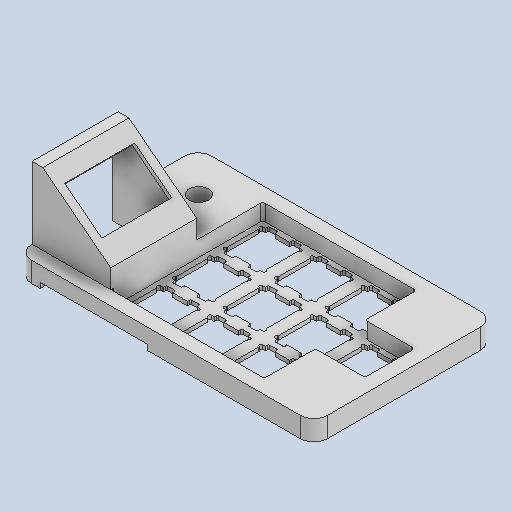
# Autodesk Inventor part: q
Saved by Autodesk Inventor 2025.2 (Build 292293000, 293)
## iProperties
Created: 2024-03-08
Part Number: q
Material: Generic
Document SubType Name: Modeling
Designer: mirun
Density: 1 g/cm^3
Appearance: Default
Author: mirun
Autodesk Inventor part; units mm, degrees
(part 1 of 2)
ref_plane "YZ Plane" through (0, 0, 0) normal (1, 0, 0) x (0, 1, 0)
sketch "Sketch1" plane through (0, 0, 0) normal (0, 1, 0) x (-1, 0, 0)
  line L0 (7.25, 5.8376) -> (7.25, -5.8376)
  line L1 (-7.25, -5.8376) -> (-7.25, 5.8376)
  line L2 (-7.25, 7.25) -> (7.25, -7.25) construction
  line L3 (7.25, 7.25) -> (-7.25, -7.25) construction
  line L4 (6.25, 7.25) -> (2.75, 7.25) construction
  line L5 (2.75, 7.35) -> (2.75, 7.95)
  line L6 (3.25, 8.45) -> (5.75, 8.45)
  line L7 (6.25, 7.95) -> (6.25, 7.35)
  arc A0 (7.4265, 6.0765) -> (7.25, 7.25) centre (7.25, 6.65) ccw
  line L8 (-7.25, 7.25) -> (2.65, 7.25)
  line L9 (6.35, 7.25) -> (7.25, 7.25)
  arc A1 (6.25, 7.35) -> (6.35, 7.25) centre (6.35, 7.35) ccw
  arc A2 (2.65, 7.25) -> (2.75, 7.35) centre (2.65, 7.35) ccw
  arc A3 (6.25, 7.95) -> (5.75, 8.45) centre (5.75, 7.95) ccw
  arc A4 (3.25, 8.45) -> (2.75, 7.95) centre (3.25, 7.95) ccw
  arc A5 (7.4265, 6.0765) -> (7.25, 5.8376) centre (7.5, 5.8376) ccw
  line L10 (0, 0) -> (3.0164, 0)
  line L11 (0, 0) -> (0, -4.9825)
  arc A6 (7.25, -5.8376) -> (7.4265, -6.0765) centre (7.5, -5.8376) ccw
  arc A7 (7.25, -7.25) -> (7.4265, -6.0765) centre (7.25, -6.65) ccw
  line L12 (6.35, -7.25) -> (7.25, -7.25)
  line L13 (7.25, -7.25) -> (-7.25, 7.25) construction
  arc A8 (6.35, -7.25) -> (6.25, -7.35) centre (6.35, -7.35) ccw
  line L14 (6.25, -7.95) -> (6.25, -7.35)
  arc A9 (5.75, -8.45) -> (6.25, -7.95) centre (5.75, -7.95) ccw
  line L15 (6.25, -7.25) -> (2.75, -7.25) construction
  line L16 (3.25, -8.45) -> (5.75, -8.45)
  arc A10 (2.75, -7.35) -> (2.65, -7.25) centre (2.65, -7.35) ccw
  line L17 (2.75, -7.35) -> (2.75, -7.95)
  arc A11 (2.75, -7.95) -> (3.25, -8.45) centre (3.25, -7.95) ccw
  line L18 (7.25, -7.25) -> (6.35, -7.25)
  arc A12 (-6.35, 7.25) -> (-6.25, 7.35) centre (-6.35, 7.35) ccw
  line L19 (-6.35, 7.25) -> (-7.25, 7.25)
  arc A13 (-7.25, 5.8376) -> (-7.4265, 6.0765) centre (-7.5, 5.8376) ccw
  arc A14 (-7.25, 7.25) -> (-7.4265, 6.0765) centre (-7.25, 6.65) ccw
  line L20 (-6.25, 7.95) -> (-6.25, 7.35)
  line L21 (-3.25, 8.45) -> (-5.75, 8.45)
  line L22 (-2.75, 7.35) -> (-2.75, 7.95)
  line L23 (-6.25, 7.25) -> (-2.75, 7.25) construction
  arc A15 (-2.75, 7.95) -> (-3.25, 8.45) centre (-3.25, 7.95) ccw
  arc A16 (-2.75, 7.35) -> (-2.65, 7.25) centre (-2.65, 7.35) ccw
  arc A17 (-5.75, 8.45) -> (-6.25, 7.95) centre (-5.75, 7.95) ccw
  line L24 (-7.25, -7.25) -> (7.25, 7.25) construction
  line L25 (-6.25, -7.25) -> (-2.75, -7.25) construction
  arc A18 (-6.25, -7.35) -> (-6.35, -7.25) centre (-6.35, -7.35) ccw
  line L26 (-2.75, -7.35) -> (-2.75, -7.95)
  line L27 (-6.25, -7.95) -> (-6.25, -7.35)
  arc A19 (-3.25, -8.45) -> (-2.75, -7.95) centre (-3.25, -7.95) ccw
  line L28 (-3.25, -8.45) -> (-5.75, -8.45)
  arc A20 (-6.25, -7.95) -> (-5.75, -8.45) centre (-5.75, -7.95) ccw
  line L29 (-6.35, -7.25) -> (-7.25, -7.25)
  line L30 (-7.25, -7.25) -> (-6.35, -7.25)
  arc A21 (-7.4265, -6.0765) -> (-7.25, -5.8376) centre (-7.5, -5.8376) ccw
  arc A22 (-7.4265, -6.0765) -> (-7.25, -7.25) centre (-7.25, -6.65) ccw
  arc A23 (-2.65, -7.25) -> (-2.75, -7.35) centre (-2.65, -7.35) ccw
  line L31 (2.65, -7.25) -> (-2.65, -7.25)
  line L32 (-6.35, -7.25) -> (-7.25, -7.25)
  line L33 (-12.65, 7.25) -> (-11.75, 7.25)
  arc A24 (-11.5735, 6.0765) -> (-11.75, 5.8376) centre (-11.5, 5.8376) ccw
  arc A25 (-11.5735, 6.0765) -> (-11.75, 7.25) centre (-11.75, 6.65) ccw
  arc A26 (-12.75, 7.35) -> (-12.65, 7.25) centre (-12.65, 7.35) ccw
  line L34 (-11.75, 5.8376) -> (-11.75, -5.8376)
  line L35 (-26.25, -5.8376) -> (-26.25, 5.8376)
  line L36 (-26.25, 7.25) -> (-11.75, -7.25) construction
  line L37 (-11.75, 7.25) -> (-26.25, -7.25) construction
  line L38 (-12.75, 7.25) -> (-16.25, 7.25) construction
  line L39 (-19, 0) -> (-15.9836, 0)
  line L40 (-25.25, 7.25) -> (-21.75, 7.25) construction
  line L41 (-26.25, 7.25) -> (-16.35, 7.25)
  line L42 (-25.35, 7.25) -> (-26.25, 7.25)
  line L43 (-11.75, -7.25) -> (-26.25, 7.25) construction
  line L44 (-26.25, -7.25) -> (-11.75, 7.25) construction
  line L45 (-19, 0) -> (-19, -4.9825)
  line L46 (-12.75, 7.95) -> (-12.75, 7.35)
  arc A27 (-12.75, 7.95) -> (-13.25, 8.45) centre (-13.25, 7.95) ccw
  line L47 (-15.75, 8.45) -> (-13.25, 8.45)
  arc A28 (-15.75, 8.45) -> (-16.25, 7.95) centre (-15.75, 7.95) ccw
  line L48 (-16.25, 7.35) -> (-16.25, 7.95)
  arc A29 (-16.35, 7.25) -> (-16.25, 7.35) centre (-16.35, 7.35) ccw
  arc A30 (-12.65, -7.25) -> (-12.75, -7.35) centre (-12.65, -7.35) ccw
  line L49 (-12.75, -7.25) -> (-16.25, -7.25) construction
  arc A31 (-16.25, -7.35) -> (-16.35, -7.25) centre (-16.35, -7.35) ccw
  line L50 (-16.25, -7.35) -> (-16.25, -7.95)
  line L51 (-16.35, -7.25) -> (-21.65, -7.25)
  arc A32 (-21.65, -7.25) -> (-21.75, -7.35) centre (-21.65, -7.35) ccw
  line L52 (-11.75, -7.25) -> (-12.65, -7.25)
  arc A33 (-11.75, -5.8376) -> (-11.5735, -6.0765) centre (-11.5, -5.8376) ccw
  arc A34 (-11.75, -7.25) -> (-11.5735, -6.0765) centre (-11.75, -6.65) ccw
  line L53 (-12.65, -7.25) -> (-11.75, -7.25)
  arc A35 (-16.25, -7.95) -> (-15.75, -8.45) centre (-15.75, -7.95) ccw
  line L54 (-15.75, -8.45) -> (-13.25, -8.45)
  arc A36 (-13.25, -8.45) -> (-12.75, -7.95) centre (-13.25, -7.95) ccw
  line L55 (-12.75, -7.95) -> (-12.75, -7.35)
  arc A37 (-25.35, 7.25) -> (-25.25, 7.35) centre (-25.35, 7.35) ccw
  arc A38 (-21.75, 7.35) -> (-21.65, 7.25) centre (-21.65, 7.35) ccw
  line L56 (-25.25, 7.95) -> (-25.25, 7.35)
  line L57 (-21.75, 7.35) -> (-21.75, 7.95)
  arc A39 (-21.75, 7.95) -> (-22.25, 8.45) centre (-22.25, 7.95) ccw
  line L58 (-22.25, 8.45) -> (-24.75, 8.45)
  arc A40 (-24.75, 8.45) -> (-25.25, 7.95) centre (-24.75, 7.95) ccw
  line L59 (-25.25, -7.25) -> (-21.75, -7.25) construction
  line L60 (-21.75, -7.35) -> (-21.75, -7.95)
  line L61 (-22.25, -8.45) -> (-24.75, -8.45)
  line L62 (-25.25, -7.95) -> (-25.25, -7.35)
  arc A41 (-25.25, -7.95) -> (-24.75, -8.45) centre (-24.75, -7.95) ccw
  arc A42 (-25.25, -7.35) -> (-25.35, -7.25) centre (-25.35, -7.35) ccw
  line L63 (-25.35, -7.25) -> (-26.25, -7.25)
  line L64 (-26.25, -7.25) -> (-25.35, -7.25)
  line L65 (-25.35, -7.25) -> (-26.25, -7.25)
  arc A43 (-26.4265, -6.0765) -> (-26.25, -5.8376) centre (-26.5, -5.8376) ccw
  arc A44 (-26.4265, -6.0765) -> (-26.25, -7.25) centre (-26.25, -6.65) ccw
  arc A45 (-22.25, -8.45) -> (-21.75, -7.95) centre (-22.25, -7.95) ccw
  arc A46 (-26.25, 7.25) -> (-26.4265, 6.0765) centre (-26.25, 6.65) ccw
  arc A47 (-26.25, 5.8376) -> (-26.4265, 6.0765) centre (-26.5, 5.8376) ccw
  line L66 (-31.65, 7.25) -> (-30.75, 7.25)
  arc A48 (-30.5735, 6.0765) -> (-30.75, 5.8376) centre (-30.5, 5.8376) ccw
  arc A49 (-30.5735, 6.0765) -> (-30.75, 7.25) centre (-30.75, 6.65) ccw
  arc A50 (-31.75, 7.35) -> (-31.65, 7.25) centre (-31.65, 7.35) ccw
  line L67 (-30.75, 5.8376) -> (-30.75, -5.8376)
  line L68 (-45.25, -5.8376) -> (-45.25, 5.8376)
  line L69 (-45.25, 7.25) -> (-30.75, -7.25) construction
  line L70 (-30.75, 7.25) -> (-45.25, -7.25) construction
  line L71 (-31.75, 7.25) -> (-35.25, 7.25) construction
  line L72 (-38, 0) -> (-34.9836, 0)
  line L73 (-44.25, 7.25) -> (-40.75, 7.25) construction
  line L74 (-45.25, 7.25) -> (-35.35, 7.25)
  line L75 (-44.35, 7.25) -> (-45.25, 7.25)
  line L76 (-30.75, -7.25) -> (-45.25, 7.25) construction
  line L77 (-45.25, -7.25) -> (-30.75, 7.25) construction
  line L78 (-38, 0) -> (-38, -4.9825)
  line L79 (-31.75, 7.95) -> (-31.75, 7.35)
  arc A51 (-31.75, 7.95) -> (-32.25, 8.45) centre (-32.25, 7.95) ccw
  line L80 (-34.75, 8.45) -> (-32.25, 8.45)
  arc A52 (-34.75, 8.45) -> (-35.25, 7.95) centre (-34.75, 7.95) ccw
  line L81 (-35.25, 7.35) -> (-35.25, 7.95)
  arc A53 (-35.35, 7.25) -> (-35.25, 7.35) centre (-35.35, 7.35) ccw
  arc A54 (-31.65, -7.25) -> (-31.75, -7.35) centre (-31.65, -7.35) ccw
  line L82 (-31.75, -7.25) -> (-35.25, -7.25) construction
  arc A55 (-35.25, -7.35) -> (-35.35, -7.25) centre (-35.35, -7.35) ccw
  line L83 (-35.25, -7.35) -> (-35.25, -7.95)
  line L84 (-35.35, -7.25) -> (-40.65, -7.25)
  arc A56 (-40.65, -7.25) -> (-40.75, -7.35) centre (-40.65, -7.35) ccw
  line L85 (-30.75, -7.25) -> (-31.65, -7.25)
  arc A57 (-30.75, -5.8376) -> (-30.5735, -6.0765) centre (-30.5, -5.8376) ccw
  arc A58 (-30.75, -7.25) -> (-30.5735, -6.0765) centre (-30.75, -6.65) ccw
  line L86 (-31.65, -7.25) -> (-30.75, -7.25)
  arc A59 (-35.25, -7.95) -> (-34.75, -8.45) centre (-34.75, -7.95) ccw
  line L87 (-34.75, -8.45) -> (-32.25, -8.45)
  arc A60 (-32.25, -8.45) -> (-31.75, -7.95) centre (-32.25, -7.95) ccw
  line L88 (-31.75, -7.95) -> (-31.75, -7.35)
  arc A61 (-44.35, 7.25) -> (-44.25, 7.35) centre (-44.35, 7.35) ccw
  arc A62 (-40.75, 7.35) -> (-40.65, 7.25) centre (-40.65, 7.35) ccw
  line L89 (-44.25, 7.95) -> (-44.25, 7.35)
  line L90 (-40.75, 7.35) -> (-40.75, 7.95)
  arc A63 (-40.75, 7.95) -> (-41.25, 8.45) centre (-41.25, 7.95) ccw
  line L91 (-41.25, 8.45) -> (-43.75, 8.45)
  arc A64 (-43.75, 8.45) -> (-44.25, 7.95) centre (-43.75, 7.95) ccw
  line L92 (-44.25, -7.25) -> (-40.75, -7.25) construction
  line L93 (-40.75, -7.35) -> (-40.75, -7.95)
  line L94 (-41.25, -8.45) -> (-43.75, -8.45)
  line L95 (-44.25, -7.95) -> (-44.25, -7.35)
  arc A65 (-44.25, -7.95) -> (-43.75, -8.45) centre (-43.75, -7.95) ccw
  arc A66 (-44.25, -7.35) -> (-44.35, -7.25) centre (-44.35, -7.35) ccw
  line L96 (-44.35, -7.25) -> (-45.25, -7.25)
  line L97 (-45.25, -7.25) -> (-44.35, -7.25)
  line L98 (-44.35, -7.25) -> (-45.25, -7.25)
  arc A67 (-45.4265, -6.0765) -> (-45.25, -5.8376) centre (-45.5, -5.8376) ccw
  arc A68 (-45.4265, -6.0765) -> (-45.25, -7.25) centre (-45.25, -6.65) ccw
  arc A69 (-41.25, -8.45) -> (-40.75, -7.95) centre (-41.25, -7.95) ccw
  arc A70 (-45.25, 7.25) -> (-45.4265, 6.0765) centre (-45.25, 6.65) ccw
  arc A71 (-45.25, 5.8376) -> (-45.4265, 6.0765) centre (-45.5, 5.8376) ccw
  line L99 (-50.65, 7.25) -> (-49.75, 7.25)
  arc A72 (-49.5735, 6.0765) -> (-49.75, 5.8376) centre (-49.5, 5.8376) ccw
  arc A73 (-49.5735, 6.0765) -> (-49.75, 7.25) centre (-49.75, 6.65) ccw
  arc A74 (-50.75, 7.35) -> (-50.65, 7.25) centre (-50.65, 7.35) ccw
  line L100 (-49.75, 5.8376) -> (-49.75, -5.8376)
  line L101 (-64.25, -5.8376) -> (-64.25, 5.8376)
  line L102 (-64.25, 7.25) -> (-49.75, -7.25) construction
  line L103 (-49.75, 7.25) -> (-64.25, -7.25) construction
  line L104 (-50.75, 7.25) -> (-54.25, 7.25) construction
  line L105 (-57, 0) -> (-53.9836, 0)
  line L106 (-63.25, 7.25) -> (-59.75, 7.25) construction
  line L107 (-64.25, 7.25) -> (-54.35, 7.25)
  line L108 (-63.35, 7.25) -> (-64.25, 7.25)
  line L109 (-49.75, -7.25) -> (-64.25, 7.25) construction
  line L110 (-64.25, -7.25) -> (-49.75, 7.25) construction
  line L111 (-57, 0) -> (-57, -4.9825)
  line L112 (-50.75, 7.95) -> (-50.75, 7.35)
  arc A75 (-50.75, 7.95) -> (-51.25, 8.45) centre (-51.25, 7.95) ccw
  line L113 (-53.75, 8.45) -> (-51.25, 8.45)
  arc A76 (-53.75, 8.45) -> (-54.25, 7.95) centre (-53.75, 7.95) ccw
  line L114 (-54.25, 7.35) -> (-54.25, 7.95)
  arc A77 (-54.35, 7.25) -> (-54.25, 7.35) centre (-54.35, 7.35) ccw
  arc A78 (-50.65, -7.25) -> (-50.75, -7.35) centre (-50.65, -7.35) ccw
  line L115 (-50.75, -7.25) -> (-54.25, -7.25) construction
  arc A79 (-54.25, -7.35) -> (-54.35, -7.25) centre (-54.35, -7.35) ccw
  line L116 (-54.25, -7.35) -> (-54.25, -7.95)
  line L117 (-54.35, -7.25) -> (-59.65, -7.25)
  arc A80 (-59.65, -7.25) -> (-59.75, -7.35) centre (-59.65, -7.35) ccw
  line L118 (-49.75, -7.25) -> (-50.65, -7.25)
  arc A81 (-49.75, -5.8376) -> (-49.5735, -6.0765) centre (-49.5, -5.8376) ccw
  arc A82 (-49.75, -7.25) -> (-49.5735, -6.0765) centre (-49.75, -6.65) ccw
  line L119 (-50.65, -7.25) -> (-49.75, -7.25)
  arc A83 (-54.25, -7.95) -> (-53.75, -8.45) centre (-53.75, -7.95) ccw
  line L120 (-53.75, -8.45) -> (-51.25, -8.45)
  arc A84 (-51.25, -8.45) -> (-50.75, -7.95) centre (-51.25, -7.95) ccw
  line L121 (-50.75, -7.95) -> (-50.75, -7.35)
  arc A85 (-63.35, 7.25) -> (-63.25, 7.35) centre (-63.35, 7.35) ccw
  arc A86 (-59.75, 7.35) -> (-59.65, 7.25) centre (-59.65, 7.35) ccw
  line L122 (-63.25, 7.95) -> (-63.25, 7.35)
  line L123 (-59.75, 7.35) -> (-59.75, 7.95)
  arc A87 (-59.75, 7.95) -> (-60.25, 8.45) centre (-60.25, 7.95) ccw
  line L124 (-60.25, 8.45) -> (-62.75, 8.45)
  arc A88 (-62.75, 8.45) -> (-63.25, 7.95) centre (-62.75, 7.95) ccw
  line L125 (-63.25, -7.25) -> (-59.75, -7.25) construction
  line L126 (-59.75, -7.35) -> (-59.75, -7.95)
  line L127 (-60.25, -8.45) -> (-62.75, -8.45)
  line L128 (-63.25, -7.95) -> (-63.25, -7.35)
  arc A89 (-63.25, -7.95) -> (-62.75, -8.45) centre (-62.75, -7.95) ccw
  arc A90 (-63.25, -7.35) -> (-63.35, -7.25) centre (-63.35, -7.35) ccw
  line L129 (-63.35, -7.25) -> (-64.25, -7.25)
  line L130 (-64.25, -7.25) -> (-63.35, -7.25)
  line L131 (-63.35, -7.25) -> (-64.25, -7.25)
  arc A91 (-64.4265, -6.0765) -> (-64.25, -5.8376) centre (-64.5, -5.8376) ccw
  arc A92 (-64.4265, -6.0765) -> (-64.25, -7.25) centre (-64.25, -6.65) ccw
  arc A93 (-60.25, -8.45) -> (-59.75, -7.95) centre (-60.25, -7.95) ccw
  arc A94 (-64.25, 7.25) -> (-64.4265, 6.0765) centre (-64.25, 6.65) ccw
  arc A95 (-64.25, 5.8376) -> (-64.4265, 6.0765) centre (-64.5, 5.8376) ccw
  line L132 (6.35, -11.75) -> (7.25, -11.75)
  arc A96 (7.4265, -12.9235) -> (7.25, -13.1624) centre (7.5, -13.1624) ccw
  arc A97 (7.4265, -12.9235) -> (7.25, -11.75) centre (7.25, -12.35) ccw
  arc A98 (6.25, -11.65) -> (6.35, -11.75) centre (6.35, -11.65) ccw
  line L133 (7.25, -13.1624) -> (7.25, -24.8376)
  line L134 (-7.25, -24.8376) -> (-7.25, -13.1624)
  line L135 (-7.25, -11.75) -> (7.25, -26.25) construction
  line L136 (7.25, -11.75) -> (-7.25, -26.25) construction
  line L137 (6.25, -11.75) -> (2.75, -11.75) construction
  line L138 (0, -19) -> (3.0164, -19)
  line L139 (-6.25, -11.75) -> (-2.75, -11.75) construction
  line L140 (-7.25, -11.75) -> (2.65, -11.75)
  line L141 (-6.35, -11.75) -> (-7.25, -11.75)
  line L142 (7.25, -26.25) -> (-7.25, -11.75) construction
  line L143 (-7.25, -26.25) -> (7.25, -11.75) construction
  line L144 (0, -19) -> (0, -23.9825)
  line L145 (6.25, -11.05) -> (6.25, -11.65)
  arc A99 (6.25, -11.05) -> (5.75, -10.55) centre (5.75, -11.05) ccw
  line L146 (3.25, -10.55) -> (5.75, -10.55)
  arc A100 (3.25, -10.55) -> (2.75, -11.05) centre (3.25, -11.05) ccw
  line L147 (2.75, -11.65) -> (2.75, -11.05)
  arc A101 (2.65, -11.75) -> (2.75, -11.65) centre (2.65, -11.65) ccw
  arc A102 (6.35, -26.25) -> (6.25, -26.35) centre (6.35, -26.35) ccw
  line L148 (6.25, -26.25) -> (2.75, -26.25) construction
  arc A103 (2.75, -26.35) -> (2.65, -26.25) centre (2.65, -26.35) ccw
  line L149 (2.75, -26.35) -> (2.75, -26.95)
  line L150 (2.65, -26.25) -> (-2.65, -26.25)
  arc A104 (-2.65, -26.25) -> (-2.75, -26.35) centre (-2.65, -26.35) ccw
  line L151 (7.25, -26.25) -> (6.35, -26.25)
  arc A105 (7.25, -24.8376) -> (7.4265, -25.0765) centre (7.5, -24.8376) ccw
  arc A106 (7.25, -26.25) -> (7.4265, -25.0765) centre (7.25, -25.65) ccw
  line L152 (6.35, -26.25) -> (7.25, -26.25)
  arc A107 (2.75, -26.95) -> (3.25, -27.45) centre (3.25, -26.95) ccw
  line L153 (3.25, -27.45) -> (5.75, -27.45)
  arc A108 (5.75, -27.45) -> (6.25, -26.95) centre (5.75, -26.95) ccw
  line L154 (6.25, -26.95) -> (6.25, -26.35)
  arc A109 (-6.35, -11.75) -> (-6.25, -11.65) centre (-6.35, -11.65) ccw
  arc A110 (-2.75, -11.65) -> (-2.65, -11.75) centre (-2.65, -11.65) ccw
  line L155 (-6.25, -11.05) -> (-6.25, -11.65)
  line L156 (-2.75, -11.65) -> (-2.75, -11.05)
  arc A111 (-2.75, -11.05) -> (-3.25, -10.55) centre (-3.25, -11.05) ccw
  line L157 (-3.25, -10.55) -> (-5.75, -10.55)
  arc A112 (-5.75, -10.55) -> (-6.25, -11.05) centre (-5.75, -11.05) ccw
  line L158 (-6.25, -26.25) -> (-2.75, -26.25) construction
  line L159 (-2.75, -26.35) -> (-2.75, -26.95)
  line L160 (-3.25, -27.45) -> (-5.75, -27.45)
  line L161 (-6.25, -26.95) -> (-6.25, -26.35)
  arc A113 (-6.25, -26.95) -> (-5.75, -27.45) centre (-5.75, -26.95) ccw
  arc A114 (-6.25, -26.35) -> (-6.35, -26.25) centre (-6.35, -26.35) ccw
  line L162 (-6.35, -26.25) -> (-7.25, -26.25)
  line L163 (-7.25, -26.25) -> (-6.35, -26.25)
  line L164 (-6.35, -26.25) -> (-7.25, -26.25)
  arc A115 (-7.4265, -25.0765) -> (-7.25, -24.8376) centre (-7.5, -24.8376) ccw
  arc A116 (-7.4265, -25.0765) -> (-7.25, -26.25) centre (-7.25, -25.65) ccw
  arc A117 (-3.25, -27.45) -> (-2.75, -26.95) centre (-3.25, -26.95) ccw
  arc A118 (-7.25, -11.75) -> (-7.4265, -12.9235) centre (-7.25, -12.35) ccw
  arc A119 (-7.25, -13.1624) -> (-7.4265, -12.9235) centre (-7.5, -13.1624) ccw
  line L165 (-12.65, -11.75) -> (-11.75, -11.75)
  arc A120 (-11.5735, -12.9235) -> (-11.75, -13.1624) centre (-11.5, -13.1624) ccw
  arc A121 (-11.5735, -12.9235) -> (-11.75, -11.75) centre (-11.75, -12.35) ccw
  arc A122 (-12.75, -11.65) -> (-12.65, -11.75) centre (-12.65, -11.65) ccw
  line L166 (-11.75, -13.1624) -> (-11.75, -24.8376)
  line L167 (-26.25, -24.8376) -> (-26.25, -13.1624)
  line L168 (-26.25, -11.75) -> (-11.75, -26.25) construction
  line L169 (-11.75, -11.75) -> (-26.25, -26.25) construction
  line L170 (-12.75, -11.75) -> (-16.25, -11.75) construction
  line L171 (-19, -19) -> (-15.9836, -19)
  line L172 (-25.25, -11.75) -> (-21.75, -11.75) construction
  line L173 (-26.25, -11.75) -> (-16.35, -11.75)
  line L174 (-25.35, -11.75) -> (-26.25, -11.75)
  line L175 (-11.75, -26.25) -> (-26.25, -11.75) construction
  line L176 (-26.25, -26.25) -> (-11.75, -11.75) construction
  line L177 (-19, -19) -> (-19, -23.9825)
  line L178 (-12.75, -11.05) -> (-12.75, -11.65)
  arc A123 (-12.75, -11.05) -> (-13.25, -10.55) centre (-13.25, -11.05) ccw
  line L179 (-15.75, -10.55) -> (-13.25, -10.55)
  arc A124 (-15.75, -10.55) -> (-16.25, -11.05) centre (-15.75, -11.05) ccw
  line L180 (-16.25, -11.65) -> (-16.25, -11.05)
  arc A125 (-16.35, -11.75) -> (-16.25, -11.65) centre (-16.35, -11.65) ccw
  arc A126 (-12.65, -26.25) -> (-12.75, -26.35) centre (-12.65, -26.35) ccw
  line L181 (-12.75, -26.25) -> (-16.25, -26.25) construction
  arc A127 (-16.25, -26.35) -> (-16.35, -26.25) centre (-16.35, -26.35) ccw
  line L182 (-16.25, -26.35) -> (-16.25, -26.95)
  line L183 (-16.35, -26.25) -> (-21.65, -26.25)
  arc A128 (-21.65, -26.25) -> (-21.75, -26.35) centre (-21.65, -26.35) ccw
  line L184 (-11.75, -26.25) -> (-12.65, -26.25)
  arc A129 (-11.75, -24.8376) -> (-11.5735, -25.0765) centre (-11.5, -24.8376) ccw
  arc A130 (-11.75, -26.25) -> (-11.5735, -25.0765) centre (-11.75, -25.65) ccw
  line L185 (-12.65, -26.25) -> (-11.75, -26.25)
  arc A131 (-16.25, -26.95) -> (-15.75, -27.45) centre (-15.75, -26.95) ccw
  line L186 (-15.75, -27.45) -> (-13.25, -27.45)
  arc A132 (-13.25, -27.45) -> (-12.75, -26.95) centre (-13.25, -26.95) ccw
  line L187 (-12.75, -26.95) -> (-12.75, -26.35)
  arc A133 (-25.35, -11.75) -> (-25.25, -11.65) centre (-25.35, -11.65) ccw
  arc A134 (-21.75, -11.65) -> (-21.65, -11.75) centre (-21.65, -11.65) ccw
  line L188 (-25.25, -11.05) -> (-25.25, -11.65)
  line L189 (-21.75, -11.65) -> (-21.75, -11.05)
  arc A135 (-21.75, -11.05) -> (-22.25, -10.55) centre (-22.25, -11.05) ccw
  line L190 (-22.25, -10.55) -> (-24.75, -10.55)
  arc A136 (-24.75, -10.55) -> (-25.25, -11.05) centre (-24.75, -11.05) ccw
  line L191 (-25.25, -26.25) -> (-21.75, -26.25) construction
  line L192 (-21.75, -26.35) -> (-21.75, -26.95)
  line L193 (-22.25, -27.45) -> (-24.75, -27.45)
  line L194 (-25.25, -26.95) -> (-25.25, -26.35)
  arc A137 (-25.25, -26.95) -> (-24.75, -27.45) centre (-24.75, -26.95) ccw
  arc A138 (-25.25, -26.35) -> (-25.35, -26.25) centre (-25.35, -26.35) ccw
  line L195 (-25.35, -26.25) -> (-26.25, -26.25)
  line L196 (-26.25, -26.25) -> (-25.35, -26.25)
  line L197 (-25.35, -26.25) -> (-26.25, -26.25)
  arc A139 (-26.4265, -25.0765) -> (-26.25, -24.8376) centre (-26.5, -24.8376) ccw
  arc A140 (-26.4265, -25.0765) -> (-26.25, -26.25) centre (-26.25, -25.65) ccw
  arc A141 (-22.25, -27.45) -> (-21.75, -26.95) centre (-22.25, -26.95) ccw
  arc A142 (-26.25, -11.75) -> (-26.4265, -12.9235) centre (-26.25, -12.35) ccw
  arc A143 (-26.25, -13.1624) -> (-26.4265, -12.9235) centre (-26.5, -13.1624) ccw
  line L198 (-31.65, -11.75) -> (-30.75, -11.75)
  arc A144 (-30.5735, -12.9235) -> (-30.75, -13.1624) centre (-30.5, -13.1624) ccw
  arc A145 (-30.5735, -12.9235) -> (-30.75, -11.75) centre (-30.75, -12.35) ccw
  arc A146 (-31.75, -11.65) -> (-31.65, -11.75) centre (-31.65, -11.65) ccw
  line L199 (-30.75, -13.1624) -> (-30.75, -24.8376)
  line L200 (-45.25, -24.8376) -> (-45.25, -13.1624)
  line L201 (-45.25, -11.75) -> (-30.75, -26.25) construction
  line L202 (-30.75, -11.75) -> (-45.25, -26.25) construction
  line L203 (-31.75, -11.75) -> (-35.25, -11.75) construction
  line L204 (-38, -19) -> (-34.9836, -19)
  line L205 (-44.25, -11.75) -> (-40.75, -11.75) construction
  line L206 (-45.25, -11.75) -> (-35.35, -11.75)
  line L207 (-44.35, -11.75) -> (-45.25, -11.75)
  line L208 (-30.75, -26.25) -> (-45.25, -11.75) construction
  line L209 (-45.25, -26.25) -> (-30.75, -11.75) construction
  line L210 (-38, -19) -> (-38, -23.9825)
  line L211 (-31.75, -11.05) -> (-31.75, -11.65)
  arc A147 (-31.75, -11.05) -> (-32.25, -10.55) centre (-32.25, -11.05) ccw
  line L212 (-34.75, -10.55) -> (-32.25, -10.55)
  arc A148 (-34.75, -10.55) -> (-35.25, -11.05) centre (-34.75, -11.05) ccw
  line L213 (-35.25, -11.65) -> (-35.25, -11.05)
  arc A149 (-35.35, -11.75) -> (-35.25, -11.65) centre (-35.35, -11.65) ccw
  arc A150 (-31.65, -26.25) -> (-31.75, -26.35) centre (-31.65, -26.35) ccw
  line L214 (-31.75, -26.25) -> (-35.25, -26.25) construction
  arc A151 (-35.25, -26.35) -> (-35.35, -26.25) centre (-35.35, -26.35) ccw
  line L215 (-35.25, -26.35) -> (-35.25, -26.95)
  line L216 (-35.35, -26.25) -> (-40.65, -26.25)
  arc A152 (-40.65, -26.25) -> (-40.75, -26.35) centre (-40.65, -26.35) ccw
  line L217 (-30.75, -26.25) -> (-31.65, -26.25)
  arc A153 (-30.75, -24.8376) -> (-30.5735, -25.0765) centre (-30.5, -24.8376) ccw
  arc A154 (-30.75, -26.25) -> (-30.5735, -25.0765) centre (-30.75, -25.65) ccw
  line L218 (-31.65, -26.25) -> (-30.75, -26.25)
  arc A155 (-35.25, -26.95) -> (-34.75, -27.45) centre (-34.75, -26.95) ccw
  line L219 (-34.75, -27.45) -> (-32.25, -27.45)
  arc A156 (-32.25, -27.45) -> (-31.75, -26.95) centre (-32.25, -26.95) ccw
  line L220 (-31.75, -26.95) -> (-31.75, -26.35)
  arc A157 (-44.35, -11.75) -> (-44.25, -11.65) centre (-44.35, -11.65) ccw
  arc A158 (-40.75, -11.65) -> (-40.65, -11.75) centre (-40.65, -11.65) ccw
  line L221 (-44.25, -11.05) -> (-44.25, -11.65)
  line L222 (-40.75, -11.65) -> (-40.75, -11.05)
  arc A159 (-40.75, -11.05) -> (-41.25, -10.55) centre (-41.25, -11.05) ccw
  line L223 (-41.25, -10.55) -> (-43.75, -10.55)
  arc A160 (-43.75, -10.55) -> (-44.25, -11.05) centre (-43.75, -11.05) ccw
  line L224 (-44.25, -26.25) -> (-40.75, -26.25) construction
  line L225 (-40.75, -26.35) -> (-40.75, -26.95)
  line L226 (-41.25, -27.45) -> (-43.75, -27.45)
  line L227 (-44.25, -26.95) -> (-44.25, -26.35)
  arc A161 (-44.25, -26.95) -> (-43.75, -27.45) centre (-43.75, -26.95) ccw
  arc A162 (-44.25, -26.35) -> (-44.35, -26.25) centre (-44.35, -26.35) ccw
  line L228 (-44.35, -26.25) -> (-45.25, -26.25)
  line L229 (-45.25, -26.25) -> (-44.35, -26.25)
  line L230 (-44.35, -26.25) -> (-45.25, -26.25)
  arc A163 (-45.4265, -25.0765) -> (-45.25, -24.8376) centre (-45.5, -24.8376) ccw
  arc A164 (-45.4265, -25.0765) -> (-45.25, -26.25) centre (-45.25, -25.65) ccw
  arc A165 (-41.25, -27.45) -> (-40.75, -26.95) centre (-41.25, -26.95) ccw
  arc A166 (-45.25, -11.75) -> (-45.4265, -12.9235) centre (-45.25, -12.35) ccw
  arc A167 (-45.25, -13.1624) -> (-45.4265, -12.9235) centre (-45.5, -13.1624) ccw
  line L231 (-50.65, -11.75) -> (-49.75, -11.75)
  arc A168 (-49.5735, -12.9235) -> (-49.75, -13.1624) centre (-49.5, -13.1624) ccw
  arc A169 (-49.5735, -12.9235) -> (-49.75, -11.75) centre (-49.75, -12.35) ccw
  arc A170 (-50.75, -11.65) -> (-50.65, -11.75) centre (-50.65, -11.65) ccw
  line L232 (-49.75, -13.1624) -> (-49.75, -24.8376)
  line L233 (-64.25, -24.8376) -> (-64.25, -13.1624)
  line L234 (-64.25, -11.75) -> (-49.75, -26.25) construction
  line L235 (-49.75, -11.75) -> (-64.25, -26.25) construction
  line L236 (-50.75, -11.75) -> (-54.25, -11.75) construction
  line L237 (-57, -19) -> (-53.9836, -19)
  line L238 (-63.25, -11.75) -> (-59.75, -11.75) construction
  line L239 (-64.25, -11.75) -> (-54.35, -11.75)
  line L240 (-63.35, -11.75) -> (-64.25, -11.75)
  line L241 (-49.75, -26.25) -> (-64.25, -11.75) construction
  line L242 (-64.25, -26.25) -> (-49.75, -11.75) construction
  line L243 (-57, -19) -> (-57, -23.9825)
  line L244 (-50.75, -11.05) -> (-50.75, -11.65)
  arc A171 (-50.75, -11.05) -> (-51.25, -10.55) centre (-51.25, -11.05) ccw
  line L245 (-53.75, -10.55) -> (-51.25, -10.55)
  arc A172 (-53.75, -10.55) -> (-54.25, -11.05) centre (-53.75, -11.05) ccw
  line L246 (-54.25, -11.65) -> (-54.25, -11.05)
  arc A173 (-54.35, -11.75) -> (-54.25, -11.65) centre (-54.35, -11.65) ccw
  arc A174 (-50.65, -26.25) -> (-50.75, -26.35) centre (-50.65, -26.35) ccw
  line L247 (-50.75, -26.25) -> (-54.25, -26.25) construction
  arc A175 (-54.25, -26.35) -> (-54.35, -26.25) centre (-54.35, -26.35) ccw
  line L248 (-54.25, -26.35) -> (-54.25, -26.95)
  line L249 (-54.35, -26.25) -> (-59.65, -26.25)
  arc A176 (-59.65, -26.25) -> (-59.75, -26.35) centre (-59.65, -26.35) ccw
  line L250 (-49.75, -26.25) -> (-50.65, -26.25)
  arc A177 (-49.75, -24.8376) -> (-49.5735, -25.0765) centre (-49.5, -24.8376) ccw
  arc A178 (-49.75, -26.25) -> (-49.5735, -25.0765) centre (-49.75, -25.65) ccw
  line L251 (-50.65, -26.25) -> (-49.75, -26.25)
  arc A179 (-54.25, -26.95) -> (-53.75, -27.45) centre (-53.75, -26.95) ccw
  line L252 (-53.75, -27.45) -> (-51.25, -27.45)
  arc A180 (-51.25, -27.45) -> (-50.75, -26.95) centre (-51.25, -26.95) ccw
  line L253 (-50.75, -26.95) -> (-50.75, -26.35)
  arc A181 (-63.35, -11.75) -> (-63.25, -11.65) centre (-63.35, -11.65) ccw
  arc A182 (-59.75, -11.65) -> (-59.65, -11.75) centre (-59.65, -11.65) ccw
  line L254 (-63.25, -11.05) -> (-63.25, -11.65)
  line L255 (-59.75, -11.65) -> (-59.75, -11.05)
  arc A183 (-59.75, -11.05) -> (-60.25, -10.55) centre (-60.25, -11.05) ccw
  line L256 (-60.25, -10.55) -> (-62.75, -10.55)
  arc A184 (-62.75, -10.55) -> (-63.25, -11.05) centre (-62.75, -11.05) ccw
  line L257 (-63.25, -26.25) -> (-59.75, -26.25) construction
  line L258 (-59.75, -26.35) -> (-59.75, -26.95)
  line L259 (-60.25, -27.45) -> (-62.75, -27.45)
  line L260 (-63.25, -26.95) -> (-63.25, -26.35)
  arc A185 (-63.25, -26.95) -> (-62.75, -27.45) centre (-62.75, -26.95) ccw
  arc A186 (-63.25, -26.35) -> (-63.35, -26.25) centre (-63.35, -26.35) ccw
  line L261 (-63.35, -26.25) -> (-64.25, -26.25)
  line L262 (-64.25, -26.25) -> (-63.35, -26.25)
  line L263 (-63.35, -26.25) -> (-64.25, -26.25)
  arc A187 (-64.4265, -25.0765) -> (-64.25, -24.8376) centre (-64.5, -24.8376) ccw
  arc A188 (-64.4265, -25.0765) -> (-64.25, -26.25) centre (-64.25, -25.65) ccw
  arc A189 (-60.25, -27.45) -> (-59.75, -26.95) centre (-60.25, -26.95) ccw
  arc A190 (-64.25, -11.75) -> (-64.4265, -12.9235) centre (-64.25, -12.35) ccw
  arc A191 (-64.25, -13.1624) -> (-64.4265, -12.9235) centre (-64.5, -13.1624) ccw
  line L264 (6.35, -30.75) -> (7.25, -30.75)
  arc A192 (7.4265, -31.9235) -> (7.25, -32.1624) centre (7.5, -32.1624) ccw
  arc A193 (7.4265, -31.9235) -> (7.25, -30.75) centre (7.25, -31.35) ccw
  arc A194 (6.25, -30.65) -> (6.35, -30.75) centre (6.35, -30.65) ccw
  line L265 (7.25, -32.1624) -> (7.25, -43.8376)
  line L266 (-7.25, -43.8376) -> (-7.25, -32.1624)
  line L267 (-7.25, -30.75) -> (7.25, -45.25) construction
  line L268 (7.25, -30.75) -> (-7.25, -45.25) construction
  line L269 (6.25, -30.75) -> (2.75, -30.75) construction
  line L270 (0, -38) -> (3.0164, -38)
  line L271 (-6.25, -30.75) -> (-2.75, -30.75) construction
  line L272 (-7.25, -30.75) -> (2.65, -30.75)
  line L273 (-6.35, -30.75) -> (-7.25, -30.75)
  line L274 (7.25, -45.25) -> (-7.25, -30.75) construction
  line L275 (-7.25, -45.25) -> (7.25, -30.75) construction
  line L276 (0, -38) -> (0, -42.9825)
  line L277 (6.25, -30.05) -> (6.25, -30.65)
  arc A195 (6.25, -30.05) -> (5.75, -29.55) centre (5.75, -30.05) ccw
  line L278 (3.25, -29.55) -> (5.75, -29.55)
  arc A196 (3.25, -29.55) -> (2.75, -30.05) centre (3.25, -30.05) ccw
  line L279 (2.75, -30.65) -> (2.75, -30.05)
  arc A197 (2.65, -30.75) -> (2.75, -30.65) centre (2.65, -30.65) ccw
  arc A198 (6.35, -45.25) -> (6.25, -45.35) centre (6.35, -45.35) ccw
  line L280 (6.25, -45.25) -> (2.75, -45.25) construction
  arc A199 (2.75, -45.35) -> (2.65, -45.25) centre (2.65, -45.35) ccw
  line L281 (2.75, -45.35) -> (2.75, -45.95)
  line L282 (2.65, -45.25) -> (-2.65, -45.25)
  arc A200 (-2.65, -45.25) -> (-2.75, -45.35) centre (-2.65, -45.35) ccw
  line L283 (7.25, -45.25) -> (6.35, -45.25)
  arc A201 (7.25, -43.8376) -> (7.4265, -44.0765) centre (7.5, -43.8376) ccw
  arc A202 (7.25, -45.25) -> (7.4265, -44.0765) centre (7.25, -44.65) ccw
  line L284 (6.35, -45.25) -> (7.25, -45.25)
  arc A203 (2.75, -45.95) -> (3.25, -46.45) centre (3.25, -45.95) ccw
  line L285 (3.25, -46.45) -> (5.75, -46.45)
  arc A204 (5.75, -46.45) -> (6.25, -45.95) centre (5.75, -45.95) ccw
  line L286 (6.25, -45.95) -> (6.25, -45.35)
  arc A205 (-6.35, -30.75) -> (-6.25, -30.65) centre (-6.35, -30.65) ccw
  arc A206 (-2.75, -30.65) -> (-2.65, -30.75) centre (-2.65, -30.65) ccw
  line L287 (-6.25, -30.05) -> (-6.25, -30.65)
  line L288 (-2.75, -30.65) -> (-2.75, -30.05)
  arc A207 (-2.75, -30.05) -> (-3.25, -29.55) centre (-3.25, -30.05) ccw
  line L289 (-3.25, -29.55) -> (-5.75, -29.55)
  arc A208 (-5.75, -29.55) -> (-6.25, -30.05) centre (-5.75, -30.05) ccw
  line L290 (-6.25, -45.25) -> (-2.75, -45.25) construction
  line L291 (-2.75, -45.35) -> (-2.75, -45.95)
  line L292 (-3.25, -46.45) -> (-5.75, -46.45)
  line L293 (-6.25, -45.95) -> (-6.25, -45.35)
  arc A209 (-6.25, -45.95) -> (-5.75, -46.45) centre (-5.75, -45.95) ccw
  arc A210 (-6.25, -45.35) -> (-6.35, -45.25) centre (-6.35, -45.35) ccw
  line L294 (-6.35, -45.25) -> (-7.25, -45.25)
  line L295 (-7.25, -45.25) -> (-6.35, -45.25)
  line L296 (-6.35, -45.25) -> (-7.25, -45.25)
  arc A211 (-7.4265, -44.0765) -> (-7.25, -43.8376) centre (-7.5, -43.8376) ccw
  arc A212 (-7.4265, -44.0765) -> (-7.25, -45.25) centre (-7.25, -44.65) ccw
  arc A213 (-3.25, -46.45) -> (-2.75, -45.95) centre (-3.25, -45.95) ccw
  arc A214 (-7.25, -30.75) -> (-7.4265, -31.9235) centre (-7.25, -31.35) ccw
  arc A215 (-7.25, -32.1624) -> (-7.4265, -31.9235) centre (-7.5, -32.1624) ccw
  line L297 (-12.65, -30.75) -> (-11.75, -30.75)
  arc A216 (-11.5735, -31.9235) -> (-11.75, -32.1624) centre (-11.5, -32.1624) ccw
  arc A217 (-11.5735, -31.9235) -> (-11.75, -30.75) centre (-11.75, -31.35) ccw
  arc A218 (-12.75, -30.65) -> (-12.65, -30.75) centre (-12.65, -30.65) ccw
  line L298 (-11.75, -32.1624) -> (-11.75, -43.8376)
  line L299 (-26.25, -43.8376) -> (-26.25, -32.1624)
  line L300 (-26.25, -30.75) -> (-11.75, -45.25) construction
  line L301 (-11.75, -30.75) -> (-26.25, -45.25) construction
  line L302 (-12.75, -30.75) -> (-16.25, -30.75) construction
  line L303 (-19, -38) -> (-15.9836, -38)
  line L304 (-25.25, -30.75) -> (-21.75, -30.75) construction
  line L305 (-26.25, -30.75) -> (-16.35, -30.75)
  line L306 (-25.35, -30.75) -> (-26.25, -30.75)
  line L307 (-11.75, -45.25) -> (-26.25, -30.75) construction
  line L308 (-26.25, -45.25) -> (-11.75, -30.75) construction
  line L309 (-19, -38) -> (-19, -42.9825)
  line L310 (-12.75, -30.05) -> (-12.75, -30.65)
  arc A219 (-12.75, -30.05) -> (-13.25, -29.55) centre (-13.25, -30.05) ccw
  line L311 (-15.75, -29.55) -> (-13.25, -29.55)
  arc A220 (-15.75, -29.55) -> (-16.25, -30.05) centre (-15.75, -30.05) ccw
  line L312 (-16.25, -30.65) -> (-16.25, -30.05)
  arc A221 (-16.35, -30.75) -> (-16.25, -30.65) centre (-16.35, -30.65) ccw
  arc A222 (-12.65, -45.25) -> (-12.75, -45.35) centre (-12.65, -45.35) ccw
  line L313 (-12.75, -45.25) -> (-16.25, -45.25) construction
  arc A223 (-16.25, -45.35) -> (-16.35, -45.25) centre (-16.35, -45.35) ccw
  line L314 (-16.25, -45.35) -> (-16.25, -45.95)
  line L315 (-16.35, -45.25) -> (-21.65, -45.25)
  arc A224 (-21.65, -45.25) -> (-21.75, -45.35) centre (-21.65, -45.35) ccw
  line L316 (-11.75, -45.25) -> (-12.65, -45.25)
  arc A225 (-11.75, -43.8376) -> (-11.5735, -44.0765) centre (-11.5, -43.8376) ccw
  arc A226 (-11.75, -45.25) -> (-11.5735, -44.0765) centre (-11.75, -44.65) ccw
  line L317 (-12.65, -45.25) -> (-11.75, -45.25)
  arc A227 (-16.25, -45.95) -> (-15.75, -46.45) centre (-15.75, -45.95) ccw
  line L318 (-15.75, -46.45) -> (-13.25, -46.45)
  arc A228 (-13.25, -46.45) -> (-12.75, -45.95) centre (-13.25, -45.95) ccw
  line L319 (-12.75, -45.95) -> (-12.75, -45.35)
  arc A229 (-25.35, -30.75) -> (-25.25, -30.65) centre (-25.35, -30.65) ccw
  arc A230 (-21.75, -30.65) -> (-21.65, -30.75) centre (-21.65, -30.65) ccw
  line L320 (-25.25, -30.05) -> (-25.25, -30.65)
  line L321 (-21.75, -30.65) -> (-21.75, -30.05)
  arc A231 (-21.75, -30.05) -> (-22.25, -29.55) centre (-22.25, -30.05) ccw
  line L322 (-22.25, -29.55) -> (-24.75, -29.55)
  arc A232 (-24.75, -29.55) -> (-25.25, -30.05) centre (-24.75, -30.05) ccw
  line L323 (-25.25, -45.25) -> (-21.75, -45.25) construction
  line L324 (-21.75, -45.35) -> (-21.75, -45.95)
  line L325 (-22.25, -46.45) -> (-24.75, -46.45)
  line L326 (-25.25, -45.95) -> (-25.25, -45.35)
  arc A233 (-25.25, -45.95) -> (-24.75, -46.45) centre (-24.75, -45.95) ccw
  arc A234 (-25.25, -45.35) -> (-25.35, -45.25) centre (-25.35, -45.35) ccw
  line L327 (-25.35, -45.25) -> (-26.25, -45.25)
  line L328 (-26.25, -45.25) -> (-25.35, -45.25)
  line L329 (-25.35, -45.25) -> (-26.25, -45.25)
  arc A235 (-26.4265, -44.0765) -> (-26.25, -43.8376) centre (-26.5, -43.8376) ccw
  arc A236 (-26.4265, -44.0765) -> (-26.25, -45.25) centre (-26.25, -44.65) ccw
  arc A237 (-22.25, -46.45) -> (-21.75, -45.95) centre (-22.25, -45.95) ccw
  arc A238 (-26.25, -30.75) -> (-26.4265, -31.9235) centre (-26.25, -31.35) ccw
  arc A239 (-26.25, -32.1624) -> (-26.4265, -31.9235) centre (-26.5, -32.1624) ccw
  line L330 (-31.65, -30.75) -> (-30.75, -30.75)
  arc A240 (-30.5735, -31.9235) -> (-30.75, -32.1624) centre (-30.5, -32.1624) ccw
  arc A241 (-30.5735, -31.9235) -> (-30.75, -30.75) centre (-30.75, -31.35) ccw
  arc A242 (-31.75, -30.65) -> (-31.65, -30.75) centre (-31.65, -30.65) ccw
  line L331 (-30.75, -32.1624) -> (-30.75, -43.8376)
  line L332 (-45.25, -43.8376) -> (-45.25, -32.1624)
  line L333 (-45.25, -30.75) -> (-30.75, -45.25) construction
  line L334 (-30.75, -30.75) -> (-45.25, -45.25) construction
  line L335 (-31.75, -30.75) -> (-35.25, -30.75) construction
  line L336 (-38, -38) -> (-34.9836, -38)
  line L337 (-44.25, -30.75) -> (-40.75, -30.75) construction
  line L338 (-45.25, -30.75) -> (-35.35, -30.75)
  line L339 (-44.35, -30.75) -> (-45.25, -30.75)
  line L340 (-30.75, -45.25) -> (-45.25, -30.75) construction
  line L341 (-45.25, -45.25) -> (-30.75, -30.75) construction
  line L342 (-38, -38) -> (-38, -42.9825)
  line L343 (-31.75, -30.05) -> (-31.75, -30.65)
  arc A243 (-31.75, -30.05) -> (-32.25, -29.55) centre (-32.25, -30.05) ccw
  line L344 (-34.75, -29.55) -> (-32.25, -29.55)
  arc A244 (-34.75, -29.55) -> (-35.25, -30.05) centre (-34.75, -30.05) ccw
  line L345 (-35.25, -30.65) -> (-35.25, -30.05)
  arc A245 (-35.35, -30.75) -> (-35.25, -30.65) centre (-35.35, -30.65) ccw
  arc A246 (-31.65, -45.25) -> (-31.75, -45.35) centre (-31.65, -45.35) ccw
  line L346 (-31.75, -45.25) -> (-35.25, -45.25) construction
  arc A247 (-35.25, -45.35) -> (-35.35, -45.25) centre (-35.35, -45.35) ccw
  line L347 (-35.25, -45.35) -> (-35.25, -45.95)
  line L348 (-35.35, -45.25) -> (-40.65, -45.25)
  arc A248 (-40.65, -45.25) -> (-40.75, -45.35) centre (-40.65, -45.35) ccw
  line L349 (-30.75, -45.25) -> (-31.65, -45.25)
  arc A249 (-30.75, -43.8376) -> (-30.5735, -44.0765) centre (-30.5, -43.8376) ccw
  arc A250 (-30.75, -45.25) -> (-30.5735, -44.0765) centre (-30.75, -44.65) ccw
  line L350 (-31.65, -45.25) -> (-30.75, -45.25)
  arc A251 (-35.25, -45.95) -> (-34.75, -46.45) centre (-34.75, -45.95) ccw
  line L351 (-34.75, -46.45) -> (-32.25, -46.45)
  arc A252 (-32.25, -46.45) -> (-31.75, -45.95) centre (-32.25, -45.95) ccw
  line L352 (-31.75, -45.95) -> (-31.75, -45.35)
  arc A253 (-44.35, -30.75) -> (-44.25, -30.65) centre (-44.35, -30.65) ccw
  arc A254 (-40.75, -30.65) -> (-40.65, -30.75) centre (-40.65, -30.65) ccw
  line L353 (-44.25, -30.05) -> (-44.25, -30.65)
  line L354 (-40.75, -30.65) -> (-40.75, -30.05)
  arc A255 (-40.75, -30.05) -> (-41.25, -29.55) centre (-41.25, -30.05) ccw
  line L355 (-41.25, -29.55) -> (-43.75, -29.55)
  arc A256 (-43.75, -29.55) -> (-44.25, -30.05) centre (-43.75, -30.05) ccw
  line L356 (-44.25, -45.25) -> (-40.75, -45.25) construction
  line L357 (-40.75, -45.35) -> (-40.75, -45.95)
  line L358 (-41.25, -46.45) -> (-43.75, -46.45)
  line L359 (-44.25, -45.95) -> (-44.25, -45.35)
  arc A257 (-44.25, -45.95) -> (-43.75, -46.45) centre (-43.75, -45.95) ccw
  arc A258 (-44.25, -45.35) -> (-44.35, -45.25) centre (-44.35, -45.35) ccw
  line L360 (-44.35, -45.25) -> (-45.25, -45.25)
  line L361 (-45.25, -45.25) -> (-44.35, -45.25)
  line L362 (-44.35, -45.25) -> (-45.25, -45.25)
  arc A259 (-45.4265, -44.0765) -> (-45.25, -43.8376) centre (-45.5, -43.8376) ccw
  arc A260 (-45.4265, -44.0765) -> (-45.25, -45.25) centre (-45.25, -44.65) ccw
  arc A261 (-41.25, -46.45) -> (-40.75, -45.95) centre (-41.25, -45.95) ccw
  arc A262 (-45.25, -30.75) -> (-45.4265, -31.9235) centre (-45.25, -31.35) ccw
  arc A263 (-45.25, -32.1624) -> (-45.4265, -31.9235) centre (-45.5, -32.1624) ccw
  line L363 (-50.65, -30.75) -> (-49.75, -30.75)
  arc A264 (-49.5735, -31.9235) -> (-49.75, -32.1624) centre (-49.5, -32.1624) ccw
  arc A265 (-49.5735, -31.9235) -> (-49.75, -30.75) centre (-49.75, -31.35) ccw
  arc A266 (-50.75, -30.65) -> (-50.65, -30.75) centre (-50.65, -30.65) ccw
  line L364 (-49.75, -32.1624) -> (-49.75, -43.8376)
  line L365 (-64.25, -43.8376) -> (-64.25, -32.1624)
  line L366 (-64.25, -30.75) -> (-49.75, -45.25) construction
  line L367 (-49.75, -30.75) -> (-64.25, -45.25) construction
  line L368 (-50.75, -30.75) -> (-54.25, -30.75) construction
  line L369 (-57, -38) -> (-53.9836, -38)
  line L370 (-63.25, -30.75) -> (-59.75, -30.75) construction
  line L371 (-64.25, -30.75) -> (-54.35, -30.75)
  line L372 (-63.35, -30.75) -> (-64.25, -30.75)
  line L373 (-49.75, -45.25) -> (-64.25, -30.75) construction
  line L374 (-64.25, -45.25) -> (-49.75, -30.75) construction
  line L375 (-57, -38) -> (-57, -42.9825)
  line L376 (-50.75, -30.05) -> (-50.75, -30.65)
  arc A267 (-50.75, -30.05) -> (-51.25, -29.55) centre (-51.25, -30.05) ccw
  line L377 (-53.75, -29.55) -> (-51.25, -29.55)
  arc A268 (-53.75, -29.55) -> (-54.25, -30.05) centre (-53.75, -30.05) ccw
  line L378 (-54.25, -30.65) -> (-54.25, -30.05)
  arc A269 (-54.35, -30.75) -> (-54.25, -30.65) centre (-54.35, -30.65) ccw
  arc A270 (-50.65, -45.25) -> (-50.75, -45.35) centre (-50.65, -45.35) ccw
  line L379 (-50.75, -45.25) -> (-54.25, -45.25) construction
  arc A271 (-54.25, -45.35) -> (-54.35, -45.25) centre (-54.35, -45.35) ccw
  line L380 (-54.25, -45.35) -> (-54.25, -45.95)
  line L381 (-54.35, -45.25) -> (-59.65, -45.25)
  arc A272 (-59.65, -45.25) -> (-59.75, -45.35) centre (-59.65, -45.35) ccw
  line L382 (-49.75, -45.25) -> (-50.65, -45.25)
  arc A273 (-49.75, -43.8376) -> (-49.5735, -44.0765) centre (-49.5, -43.8376) ccw
  arc A274 (-49.75, -45.25) -> (-49.5735, -44.0765) centre (-49.75, -44.65) ccw
  line L383 (-50.65, -45.25) -> (-49.75, -45.25)
  arc A275 (-54.25, -45.95) -> (-53.75, -46.45) centre (-53.75, -45.95) ccw
  line L384 (-53.75, -46.45) -> (-51.25, -46.45)
  arc A276 (-51.25, -46.45) -> (-50.75, -45.95) centre (-51.25, -45.95) ccw
  line L385 (-50.75, -45.95) -> (-50.75, -45.35)
  arc A277 (-63.35, -30.75) -> (-63.25, -30.65) centre (-63.35, -30.65) ccw
  arc A278 (-59.75, -30.65) -> (-59.65, -30.75) centre (-59.65, -30.65) ccw
  line L386 (-63.25, -30.05) -> (-63.25, -30.65)
  line L387 (-59.75, -30.65) -> (-59.75, -30.05)
  arc A279 (-59.75, -30.05) -> (-60.25, -29.55) centre (-60.25, -30.05) ccw
  line L388 (-60.25, -29.55) -> (-62.75, -29.55)
  arc A280 (-62.75, -29.55) -> (-63.25, -30.05) centre (-62.75, -30.05) ccw
  line L389 (-63.25, -45.25) -> (-59.75, -45.25) construction
  line L390 (-59.75, -45.35) -> (-59.75, -45.95)
  line L391 (-60.25, -46.45) -> (-62.75, -46.45)
  line L392 (-63.25, -45.95) -> (-63.25, -45.35)
  arc A281 (-63.25, -45.95) -> (-62.75, -46.45) centre (-62.75, -45.95) ccw
  arc A282 (-63.25, -45.35) -> (-63.35, -45.25) centre (-63.35, -45.35) ccw
  line L393 (-63.35, -45.25) -> (-64.25, -45.25)
  line L394 (-64.25, -45.25) -> (-63.35, -45.25)
  line L395 (-63.35, -45.25) -> (-64.25, -45.25)
  arc A283 (-64.4265, -44.0765) -> (-64.25, -43.8376) centre (-64.5, -43.8376) ccw
  arc A284 (-64.4265, -44.0765) -> (-64.25, -45.25) centre (-64.25, -44.65) ccw
  arc A285 (-60.25, -46.45) -> (-59.75, -45.95) centre (-60.25, -45.95) ccw
  arc A286 (-64.25, -30.75) -> (-64.4265, -31.9235) centre (-64.25, -31.35) ccw
  arc A287 (-64.25, -32.1624) -> (-64.4265, -31.9235) centre (-64.5, -32.1624) ccw
  line L396 (-76.5, -56.5) -> (38.5, -56.5)
  line L397 (38.5, -56.5) -> (38.5, 18.5)
  line L398 (38.5, 18.5) -> (-76.5, 18.5)
  line L399 (-76.5, 18.5) -> (-76.5, -56.5)
  line L400 (-76.5, -56.5) -> (38.5, 18.5) construction
  line L401 (38.5, -56.5) -> (-76.5, 18.5) construction
  line L402 (-76.5, 14.5) -> (38.5, 14.5)
  line L403 (-71.52, 18.5) -> (-71.52, -56.5)
  line L404 (-64.25, -32.1624) -> (-64.25, -43.8376)
  line L405 (-76.5, -52.5) -> (38.5, -52.5)
  point P0 (2.75, 8.45)
  point P1 (6.25, 8.45)
  point P2 (6.25, 7.65)
  point P3 (7.25, 6.05)
  point P4 (7.25, -6.05)
  point P5 (6.25, -7.65)
  point P6 (6.25, -8.45)
  point P7 (2.75, -8.45)
  point P8 (-7.25, 6.05)
  point P9 (-6.25, 8.45)
  point P10 (-6.25, 7.65)
  point P11 (-2.75, 8.45)
  point P12 (-2.75, -8.45)
  point P13 (-6.25, -8.45)
  point P14 (-7.25, -6.05)
  point P15 (-6.25, -7.65)
  point P16 (-7.1278, 7.1889)
  point P17 (-6.2278, 7.1889)
  point P18 (-2.5278, 7.1889)
  point P19 (-11.75, 6.05)
  point P20 (-19, 0)
  point P21 (-12.75, 8.45)
  point P22 (-12.75, 7.65)
  point P23 (-16.25, 8.45)
  point P24 (-16.25, -8.45)
  point P25 (-11.75, -6.05)
  point P26 (-12.75, -7.65)
  point P27 (-12.75, -8.45)
  point P28 (-25.25, 7.65)
  point P29 (-25.25, 8.45)
  point P30 (-21.75, 8.45)
  point P31 (-21.75, -8.45)
  point P32 (-25.25, -8.45)
  point P33 (-25.25, -7.65)
  point P34 (-26.25, -6.05)
  point P35 (-26.25, 6.05)
  point P36 (-30.75, 6.05)
  point P37 (-38, 0)
  point P38 (-31.75, 8.45)
  point P39 (-31.75, 7.65)
  point P40 (-35.25, 8.45)
  point P41 (-35.25, -8.45)
  point P42 (-30.75, -6.05)
  point P43 (-31.75, -7.65)
  point P44 (-31.75, -8.45)
  point P45 (-44.25, 7.65)
  point P46 (-44.25, 8.45)
  point P47 (-40.75, 8.45)
  point P48 (-40.75, -8.45)
  point P49 (-44.25, -8.45)
  point P50 (-44.25, -7.65)
  point P51 (-45.25, -6.05)
  point P52 (-45.25, 6.05)
  point P53 (-49.75, 6.05)
  point P54 (-57, 0)
  point P55 (-50.75, 8.45)
  point P56 (-50.75, 7.65)
  point P57 (-54.25, 8.45)
  point P58 (-54.25, -8.45)
  point P59 (-49.75, -6.05)
  point P60 (-50.75, -7.65)
  point P61 (-50.75, -8.45)
  point P62 (-63.25, 7.65)
  point P63 (-63.25, 8.45)
  point P64 (-59.75, 8.45)
  point P65 (-59.75, -8.45)
  point P66 (-63.25, -8.45)
  point P67 (-63.25, -7.65)
  point P68 (-64.25, -6.05)
  point P69 (-64.25, 6.05)
  point P70 (7.25, -12.95)
  point P71 (0, -19)
  point P72 (6.25, -10.55)
  point P73 (6.25, -11.35)
  point P74 (2.75, -10.55)
  point P75 (2.75, -27.45)
  point P76 (7.25, -25.05)
  point P77 (6.25, -26.65)
  point P78 (6.25, -27.45)
  point P79 (-6.25, -11.35)
  point P80 (-6.25, -10.55)
  point P81 (-2.75, -10.55)
  point P82 (-2.75, -27.45)
  point P83 (-6.25, -27.45)
  point P84 (-6.25, -26.65)
  point P85 (-7.25, -25.05)
  point P86 (-7.25, -12.95)
  point P87 (-11.75, -12.95)
  point P88 (-19, -19)
  point P89 (-12.75, -10.55)
  point P90 (-12.75, -11.35)
  point P91 (-16.25, -10.55)
  point P92 (-16.25, -27.45)
  point P93 (-11.75, -25.05)
  point P94 (-12.75, -26.65)
  point P95 (-12.75, -27.45)
  point P96 (-25.25, -11.35)
  point P97 (-25.25, -10.55)
  point P98 (-21.75, -10.55)
  point P99 (-21.75, -27.45)
  point P100 (-25.25, -27.45)
  point P101 (-25.25, -26.65)
  point P102 (-26.25, -25.05)
  point P103 (-26.25, -12.95)
  point P104 (-30.75, -12.95)
  point P105 (-38, -19)
  point P106 (-31.75, -10.55)
  point P107 (-31.75, -11.35)
  point P108 (-35.25, -10.55)
  point P109 (-35.25, -27.45)
  point P110 (-30.75, -25.05)
  point P111 (-31.75, -26.65)
  point P112 (-31.75, -27.45)
  point P113 (-44.25, -11.35)
  point P114 (-44.25, -10.55)
  point P115 (-40.75, -10.55)
  point P116 (-40.75, -27.45)
  point P117 (-44.25, -27.45)
  point P118 (-44.25, -26.65)
  point P119 (-45.25, -25.05)
  point P120 (-45.25, -12.95)
  point P121 (-49.75, -12.95)
  point P122 (-57, -19)
  point P123 (-50.75, -10.55)
  point P124 (-50.75, -11.35)
  point P125 (-54.25, -10.55)
  point P126 (-54.25, -27.45)
  point P127 (-49.75, -25.05)
  point P128 (-50.75, -26.65)
  point P129 (-50.75, -27.45)
  point P130 (-63.25, -11.35)
  point P131 (-63.25, -10.55)
  point P132 (-59.75, -10.55)
  point P133 (-59.75, -27.45)
  point P134 (-63.25, -27.45)
  point P135 (-63.25, -26.65)
  point P136 (-64.25, -25.05)
  point P137 (-64.25, -12.95)
  point P138 (7.25, -31.95)
  point P139 (0, -38)
  point P140 (6.25, -29.55)
  point P141 (6.25, -30.35)
  point P142 (2.75, -29.55)
  point P143 (2.75, -46.45)
  point P144 (7.25, -44.05)
  point P145 (6.25, -45.65)
  point P146 (6.25, -46.45)
  point P147 (-6.25, -30.35)
  point P148 (-6.25, -29.55)
  point P149 (-2.75, -29.55)
  point P150 (-2.75, -46.45)
  point P151 (-6.25, -46.45)
  point P152 (-6.25, -45.65)
  point P153 (-7.25, -44.05)
  point P154 (-7.25, -31.95)
  point P155 (-11.75, -31.95)
  point P156 (-19, -38)
  point P157 (-12.75, -29.55)
  point P158 (-12.75, -30.35)
  point P159 (-16.25, -29.55)
  point P160 (-16.25, -46.45)
  point P161 (-11.75, -44.05)
  point P162 (-12.75, -45.65)
  point P163 (-12.75, -46.45)
  point P164 (-25.25, -30.35)
  point P165 (-25.25, -29.55)
  point P166 (-21.75, -29.55)
  point P167 (-21.75, -46.45)
  point P168 (-25.25, -46.45)
  point P169 (-25.25, -45.65)
  point P170 (-26.25, -44.05)
  point P171 (-26.25, -31.95)
  point P172 (-30.75, -31.95)
  point P173 (-31.75, -29.55)
  point P174 (-31.75, -30.35)
  point P175 (-35.25, -29.55)
  point P176 (-35.25, -46.45)
  point P177 (-30.75, -44.05)
  point P178 (-31.75, -45.65)
  point P179 (-31.75, -46.45)
  point P180 (-44.25, -30.35)
  point P181 (-44.25, -29.55)
  point P182 (-40.75, -29.55)
  point P183 (-40.75, -46.45)
  point P184 (-44.25, -46.45)
  point P185 (-44.25, -45.65)
  point P186 (-45.25, -44.05)
  point P187 (-45.25, -31.95)
  point P188 (-49.75, -31.95)
  point P189 (-57, -38)
  point P190 (-50.75, -29.55)
  point P191 (-50.75, -30.35)
  point P192 (-54.25, -29.55)
  point P193 (-54.25, -46.45)
  point P194 (-49.75, -44.05)
  point P195 (-50.75, -45.65)
  point P196 (-50.75, -46.45)
  point P197 (-63.25, -30.35)
  point P198 (-63.25, -29.55)
  point P199 (-59.75, -29.55)
  dimension "d0" = 14.5
  dimension "d1" = 14.5
  dimension "d2" = 3.5
  dimension "d3" = 1.2
  dimension "d4" = 1
  dimension "d5" = 1.2
  dimension "d6" = 0.1
  dimension "d7" = 0.1
  dimension "d8" = 0.5
  dimension "d9" = 0.25
  dimension "d15" = 19
  dimension "d18" = 19
  dimension "d21" = 115
  dimension "d22" = 75
  dimension "d82" = 4
  dimension "d83" = 7.27
  constraints: 812 end point, 624 point on circle, 376 point on line, 288 centre point, 70 symmetric about line, 29 midpoint, 12 tangent, 11 parallel, 7 perpendicular, 6 horizontal, 2 collinear, 1 coincident, 1 equal radius, 1 vertical, 1721 other
  measures "d0" distance of L2.end L3.end
  measures "d1" distance of L3.start L2.end
  measures "d2" distance of point (2.75, 8.45) point (6.25, 8.45)
  measures "d3" distance of L4.end point (2.75, 8.45)
  measures "d4" distance from line of L0 point (6.25, 7.65)
  measures "d5" diameter of A0
  measures "d6" radius of A1
  measures "d7" radius of A2
  measures "d8" radius of A3
  measures "d9" radius of A5
  measures "d15" distance of L9.start L33.start
  measures "d18" distance of L9.start L132.start
  measures "d21" distance of L398.end L397.end
  measures "d22" distance of L397.end L396.end
  measures "d82" distance between parallel lines of L398 L402
  measures "d83" distance between parallel lines of L403 L101